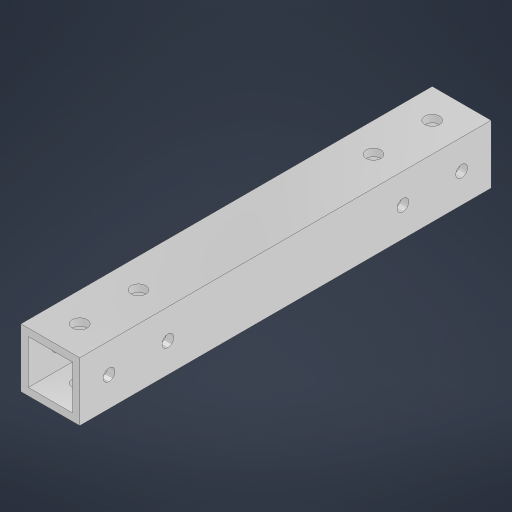
# Autodesk Inventor part: testRoboRescue_Chassis_Frame_lengthBar
Saved by Autodesk Inventor 2023 (Build 270158000, 158)
## iProperties
Created: 2022-03-14
Part Number: testRoboRescue_Chassis_Frame_lengthBar
Material: Aluminum 6061
Document SubType Name: Modeling
Designer: Nebil Oumer
Density: 2.7 g/cm^3
Appearance: Aluminum - Polished
Mass: 182.511 g
Surface Area: 434.677 cm^2
Volume: 67.5966 cm^3
Author: Nebil Oumer
Autodesk Inventor part; units mm, degrees
ref_plane "YZ Plane" through (0, 0, 0) normal (1, 0, 0) x (0, 1, 0)
ref_plane "XZ Plane" through (0, 0, 0) normal (0, 1, 0) x (-1, 0, 0)
ref_plane "XY Plane" through (0, 0, 0) normal (0, 0, 1) x (1, 0, 0)
sketch "Sketch1" plane through (0, 0, 0) normal (0, 0, 1) x (1, 0, 0)
  line L0 (0, 0) -> (25.4, 0)
  line L1 (25.4, 0) -> (25.4, 25.4)
  line L2 (25.4, 25.4) -> (0, 25.4)
  line L3 (0, 25.4) -> (0, 0)
  line L4 (22.225, 22.225) -> (22.225, 3.175)
  line L5 (22.225, 3.175) -> (3.175, 3.175)
  line L6 (3.175, 3.175) -> (3.175, 22.225)
  line L7 (3.175, 22.225) -> (22.225, 22.225)
  dimension "d0" = 25.4
  dimension "d1" = 25.4
  dimension "d2" = 3.175
  constraints: 16 end point, 4 parallel, 2 perpendicular, 1 horizontal, 3 other
  measures "d0" distance of L2.end L1.end
  measures "d1" distance of L0.end L1.end
  measures "d2" distance between parallel lines of L1 L4
extrude "Extrusion1" add sketch "Sketch1" along normal blind 177.8
sketch "Sketch2" plane through (0, 25.4, 0) normal (0, 1, 0) x (1, 0, 0)
  line L0 (25.4, 0) -> (25.4, -177.8) projected
  line L1 (25.4, -177.8) -> (0, -177.8) projected
  line L2 (25.4, 0) -> (0, 0) projected
  line L3 (0, 0) -> (0, -177.8) projected
  point P0 (12.7, -165.1)
  point P1 (12.7, -12.7)
  dimension "d5" = 12.7
  dimension "d6" = 12.7
  dimension "d7" = 12.7
  dimension "d8" = 12.7
  measures "d5" distance from line of L0 point (12.7, -165.1)
  measures "d6" distance from line of L1 point (12.7, -165.1)
  measures "d7" distance from line of L2 point (12.7, -12.7)
  measures "d8" distance from line of L3 point (12.7, -12.7)
hole "Hole1" at (12.7, 25.4, 165.1) at (12.7, 25.4, 12.7) direction (0, -1, 0) diameter 6.35 end through all
pattern_linear "Rectangular Pattern1" count 2 spacing 25.4 along (0, 0, 1) count 2 spacing 25.4 along (0, 0, -1) of "Hole1"
sketch "Sketch4" plane through (25.4, 0, 0) normal (1, 0, 0) x (0, 0, -1)
  line L0 (0, 25.4) -> (-177.8, 25.4) projected
  line L1 (-177.8, 0) -> (-177.8, 25.4) projected
  line L2 (0, 0) -> (0, 25.4) projected
  point P0 (-165.1, 12.7)
  point P1 (-12.7, 12.7)
  dimension "d31" = 12.7
  dimension "d32" = 12.7
  dimension "d33" = 12.7
  dimension "d34" = 12.7
  measures "d31" distance from line of L0 point (-165.1, 12.7)
  measures "d32" distance from line of L1 point (-165.1, 12.7)
  measures "d33" distance from line of L0 point (-12.7, 12.7)
  measures "d34" distance from line of L2 point (-12.7, 12.7)
hole "Hole3" at (25.4, 12.7, 165.1) at (25.4, 12.7, 12.7) direction (-1, 0, 0) diameter 5.08 end through all
pattern_linear "Rectangular Pattern2" count 2 spacing 25.4 along (0, 0, -1) count 2 spacing 25.4 along (0, 0, 1) of "Hole3"
equation "\"d0\" = d1"
body "Solid1"
